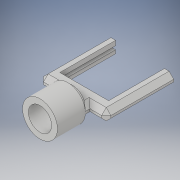
# Autodesk Inventor part: 6 Kamerahalterung
Saved by Autodesk Inventor 2018.3 (Build 223284000, 284)
## iProperties
Created: 2018-11-08
Part Number: 6 Kamerahalterung
Material: Generisch
Document SubType Name: Modeling
Designer: pgmadmin
Density: 1 g/cm^3
Appearance: Vorgabe
Author: pgmadmin
Autodesk Inventor part; units mm, degrees
ref_plane "YZ Plane" through (0, 0, 0) normal (1, 0, 0) x (0, 1, 0)
ref_plane "XZ Plane" through (0, 0, 0) normal (0, 1, 0) x (-1, 0, 0)
ref_plane "XY Plane" through (0, 0, 0) normal (0, 0, 1) x (1, 0, 0)
sketch "Skizze1" plane through (0, 0, 0) normal (0, 0, 1) x (1, 0, 0)
  line L0 (0, 0) -> (25, 0)
  line L1 (25, 0) -> (25, 24)
  line L2 (0, 24) -> (0, 0)
  line L3 (0, 24) -> (-5, 24)
  line L4 (-5, 24) -> (-5, -5)
  line L5 (-5, -5) -> (30, -5)
  line L6 (30, -5) -> (30, 24)
  line L7 (30, 24) -> (25, 24)
  constraints: 16 end point, 5 perpendicular, 2 horizontal, 1 parallel, 1 point on line
extrude "Extrusion1" add sketch "Skizze1" along normal blind 12
sketch "Skizze2" plane through (0, 0, 0) normal (0, 0, -1) x (-1, 0, 0)
  line L0 (-25, 24) -> (-23, 24)
  line L1 (-23, 24) -> (-23, -1.0226)
  line L2 (-23, -1.0226) -> (-25, -1.0226)
  line L3 (-25, -1.0226) -> (-25, 24)
  line L4 (0, 0) -> (0, 24) projected
  line L5 (0, 24) -> (-2, 24)
  line L6 (-2, 24) -> (-2, -3.2856)
  line L7 (-2, -3.2856) -> (0, -3.2856)
  line L8 (0, -3.2856) -> (0, 24)
  dimension "d7" = 2
  dimension "d8" = 2
  constraints: 16 end point, 4 parallel, 2 horizontal, 2 perpendicular
  measures "d7" distance of L1.end L2.end
  measures "d8" distance of L7.end L6.end
extrude "Extrusion2" add sketch "Skizze2" against normal blind 3
sketch "Skizze3" plane through (0, 0, 12) normal (0, 0, 1) x (1, 0, 0)
  line L0 (0, 24) -> (-5, 24) projected
  line L1 (0, 24) -> (2, 24)
  line L2 (2, 24) -> (2, -1.1552)
  line L3 (2, -1.1552) -> (0, -1.1552)
  line L4 (0, -1.1552) -> (0, 24)
  line L5 (25, 24) -> (23, 24)
  line L6 (23, 24) -> (23, -1.1552)
  line L7 (23, -1.1552) -> (25, -1.1552)
  line L8 (25, -1.1552) -> (25, 24)
  point P0 (0, 0)
  constraints: 16 end point, 4 parallel, 2 horizontal, 2 perpendicular, 1 point on line
extrude "Extrusion3" add sketch "Skizze3" against normal blind 8
sketch "Skizze4" plane through (-5, 24, 12) normal (0, 1, 0) x (1, 0, 0)
  line L0 (7, 12) -> (7, 9) projected
  line L1 (3, 11) -> (3, 6)
  line L2 (3, 6) -> (32, 6)
  line L3 (7, 8) -> (7, 0) projected
  line L4 (32, 6) -> (32, 11)
  line L5 (5, 9) -> (5, 8) projected
  line L6 (30, 9) -> (30, 8) projected
  line L7 (5, 8) -> (7, 8) projected
  line L8 (3, 11) -> (32, 11)
  line L9 (7, 9) -> (5, 9) projected
  line L10 (0, 12) -> (0, 0) projected
  line L11 (35, 0) -> (28, 0) projected
  line L12 (0, 12) -> (35, 12)
  line L13 (35, 12) -> (35, 0)
  line L14 (35, 0) -> (0, 0)
  line L15 (0, 0) -> (0, 12)
  point P0 (5, 12)
  dimension "d16" = 2
  constraints: 16 end point, 3 perpendicular, 2 horizontal, 2 parallel
  measures "d16" distance between parallel lines of L8 L9
extrude "Extrusion4" cut sketch "Skizze4" against normal blind 90.5 contours L12 L13 L11 L14 L3 L2 L4 L8 L0 | L0 L8 L1 L2 L3 L14 L10 L12
sketch "Skizze5" plane through (23, 24, 3) normal (0, 1, 0) x (1, 0, 0)
  line L0 (2.5, -1) -> (-23.5, -1)
  line L1 (-23.5, -1) -> (-23.5, 0.5)
  line L2 (-23.5, 0.5) -> (2.5, 0.5)
  line L3 (2.5, 0.5) -> (2.5, -1)
  line L4 (2, 0) -> (2, -1) projected
  line L5 (-23, 0) -> (-23, -1) projected
  point P0 (-23, 3)
  dimension "d19" = 26
  dimension "d20" = 1.5
  dimension "d21" = 0.5
  dimension "d22" = 0.5
  constraints: 8 end point, 2 parallel, 1 horizontal, 1 perpendicular
  measures "d19" distance of L1.end L2.end
  measures "d20" distance of L0.end L1.end
  measures "d21" distance between parallel lines of L4 L3
  measures "d22" distance between parallel lines of L1 L5
extrude "Extrusion5" cut sketch "Skizze5" against normal blind 24
sketch "Skizze6" plane through (-2, -5, 6) normal (0, -1, 0) x (1, 0, 0)
  circle A0 centre (14.5, -2.5) radius 7.5
  line L0 (29, 0) -> (0, 0) projected
  point P0 (2, -6)
  dimension "d25" = 15
  dimension "d26" = 2.5
  constraints: 1 centre point
  measures "d25" diameter of A0
  measures "d26" distance from line of L0 A0.centre
extrude "Extrusion6" add sketch "Skizze6" along normal blind 14
chamfer "Fase2" distance 2 angle 45 2 edges at (12.5, -5, 11) (12.5, -5, -4)
chamfer "Fase3" distance 2 angle 45 12 edges at (-2, 9.5, 1) (-2, 9.5, 6) (27, 9.5, 6) (23.2855, -5, 6) (1.7145, -5, 6) (5.4289, -6, 6) (19.5711, -6, 6) (5.4289, -6, 1) (19.5711, -6, 1) (27, 9.5, 1) (27, -5, 3.5) (-2, -5, 3.5)
chamfer "Fase4" distance 2 angle 45 4 edges at (22.2855, -5, 1) (18.5711, -5, 1) (6.4289, -5, 1) (2.7145, -5, 1)
sketch "Skizze7" plane through (12.5, -19, 3.5) normal (0, -1, 0) x (1, 0, 0)
  circle A0 centre (0, 0) radius 5
  point P0 (-12.5, -3.5)
  dimension "d42" = 10
  constraints: 1 centre point
  measures "d42" diameter of A0
extrude "Extrusion7" cut sketch "Skizze7" against normal blind 10
